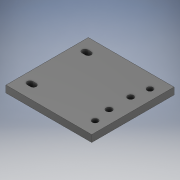
# Autodesk Inventor part: X-Axis_End_Plate_LM3004
Saved by Autodesk Inventor 2020.2 (Build 242310000, 310)
## iProperties
Created: 2019-11-14
Part Number: X-Axis_End_Plate_LM3004
Material: Polycarbonate, Smoke
Document SubType Name: Modeling
Designer: Richard Hall
Density: 1.2 g/cm^3
Appearance: Smooth - Black
Author: Richard Hall
Autodesk Inventor part; units mm, degrees
ref_plane "YZ Plane" through (0, 0, 0) normal (1, 0, 0) x (0, 1, 0)
ref_plane "XZ Plane" through (0, 0, 0) normal (0, 1, 0) x (-1, 0, 0)
ref_plane "XY Plane" through (0, 0, 0) normal (0, 0, 1) x (1, 0, 0)
sketch "Sketch1" plane through (0, 0, 0) normal (0, 1, 0) x (-1, 0, 0)
  line L0 (39.6875, -38.1) -> (-39.6875, -38.1)
  line L1 (-39.6875, -38.1) -> (-39.6875, 38.1)
  line L2 (-39.6875, 38.1) -> (39.6875, 38.1)
  line L3 (39.6875, 38.1) -> (39.6875, -38.1)
  line L4 (39.6875, -38.1) -> (-39.6875, 38.1) construction
  line L5 (-39.6875, -38.1) -> (39.6875, 38.1) construction
  point P0 (0, 0)
  dimension "d0" = 76.2
  dimension "d1" = 79.375
  constraints: 12 end point, 2 midpoint, 2 parallel, 1 horizontal, 1 perpendicular
  measures "d0" distance of L0.end L1.end
  measures "d1" distance of L0.start L0.end
extrude "Extrusion1" add sketch "Sketch1" along normal mid plane 6.35
sketch "Sketch2" plane through (0, 3.175, 0) normal (0, 1, 0) x (1, 0, 0)
  line L0 (-39.6875, 38.1) -> (-39.6875, -38.1) projected
  line L1 (39.6875, -38.1) -> (39.6875, 38.1) projected
  line L2 (39.6875, 38.1) -> (-39.6875, 38.1) projected
  line L3 (-39.6875, -38.1) -> (39.6875, -38.1) projected
  point P0 (0, 0)
  point P1 (-30.1625, 25.4)
  point P2 (-30.1625, -25.4)
  point P3 (30.1625, 25.4)
  point P4 (30.1625, -25.4)
  dimension "d4" = 9.525
  dimension "d5" = 9.525
  dimension "d6" = 9.525
  dimension "d7" = 9.525
  dimension "d8" = 12.7
  dimension "d9" = 12.7
  dimension "d10" = 12.7
  dimension "d11" = 12.7
  measures "d4" distance from line of L0 point (-30.163, 25.4)
  measures "d5" distance from line of L1 point (30.162, 25.4)
  measures "d6" distance from line of L1 point (30.162, -25.4)
  measures "d7" distance from line of L0 point (-30.162, -25.4)
  measures "d8" distance from line of L2 point (-30.163, 25.4)
  measures "d9" distance from line of L2 point (30.162, 25.4)
  measures "d10" distance from line of L3 point (-30.162, -25.4)
  measures "d11" distance from line of L3 point (30.162, -25.4)
hole "Hole1" at (-30.1625, 3.175, -25.4) at (-30.1625, 3.175, 25.4) at (30.1625, 3.175, -25.4) at (30.1625, 3.175, 25.4) direction (0, -1, 0) diameter 5.3086 end through all clearance for "Socket Head Cap Screw" size "M5" standard "Ansi Metric M Profile"
sketch "Sketch3" plane through (0, 3.175, 0) normal (0, 1, 0) x (1, 0, 0)
  circle A0 centre (30.1625, 25.4) radius 2.6543 projected
  circle A1 centre (-30.1625, 25.4) radius 2.6543 projected
  circle A2 centre (-30.1625, -25.4) radius 2.6543 projected
  circle A3 centre (30.1625, -25.4) radius 2.6543 projected
  line L0 (39.6875, -38.1) -> (39.6875, 38.1) projected
  line L1 (39.6875, 38.1) -> (-39.6875, 38.1) projected
  line L2 (-39.6875, 38.1) -> (-39.6875, -38.1) projected
  line L3 (-39.6875, -38.1) -> (39.6875, -38.1) projected
  line L4 (-30.1625, 25.4) -> (-26.9875, 25.4) construction
  line L5 (-30.1625, 22.7457) -> (-26.9875, 22.7457)
  line L6 (-26.9875, 28.0543) -> (-30.1625, 28.0543)
  arc A4 (-30.1625, 28.0543) -> (-30.1625, 22.7457) centre (-30.1625, 25.4) ccw
  arc A5 (-26.9875, 22.7457) -> (-26.9875, 28.0543) centre (-26.9875, 25.4) ccw
  line L7 (-30.1625, -25.4) -> (-26.9875, -25.4) construction
  line L8 (-30.1625, -22.7457) -> (-26.9875, -22.7457)
  line L9 (-26.9875, -28.0543) -> (-30.1625, -28.0543)
  arc A6 (-30.1625, -22.7457) -> (-30.1625, -28.0543) centre (-30.1625, -25.4) ccw
  arc A7 (-26.9875, -28.0543) -> (-26.9875, -22.7457) centre (-26.9875, -25.4) ccw
  point P0 (0, 0)
  point P1 (-28.575, 25.4)
  point P2 (-28.575, -25.4)
  dimension "d19" = 3.175
  dimension "d20" = 3.175
  constraints: 16 end point, 8 point on circle, 8 tangent, 4 centre point, 2 concentric, 2 horizontal, 2 midpoint, 2 parallel
  measures "d19" distance of L7.start L7.end
  measures "d20" distance of L4.start L4.end
extrude "Extrusion2" cut sketch "Sketch3" against normal blind 6.35 contours A1 L6 A5 L5 | A2 L8 A7 L9
sketch "Sketch4" plane through (0, 3.175, 0) normal (0, 1, 0) x (1, 0, 0)
  line L0 (39.6875, -38.1) -> (39.6875, 38.1) projected
  line L1 (39.6875, 38.1) -> (-39.6875, 38.1) projected
  line L2 (-39.6875, -38.1) -> (39.6875, -38.1) projected
  circle A0 centre (30.1625, 25.4) radius 2.6543 projected
  circle A1 centre (30.1625, -25.4) radius 2.6543 projected
  point P0 (0, 0)
  point P1 (27.6625, 10)
  point P2 (27.6625, -10)
  dimension "d33" = 15.4
  dimension "d34" = 2.5
  dimension "d35" = 15.4
  constraints: 1 vertical alignment
  measures "d33" vertical distance of point (27.662, 10) A0.centre
  measures "d34" horizontal distance of A0.centre point (27.662, 10)
  measures "d35" vertical distance of point (27.662, -10) A1.centre
hole "Hole2" at (27.6625, 3.175, -10) at (27.6625, 3.175, 10) direction (0, -1, 0) diameter 5.5 end through all
equation "\"d5\" = d4"
equation "\"d6\" = d5"
equation "\"d7\" = d4"
equation "\"d9\" = d8"
equation "\"d10\" = d8"
equation "\"d11\" = d10"
equation "\"d20\" = d19"
equation "\"d35\" = d33"
body "Solid1"
